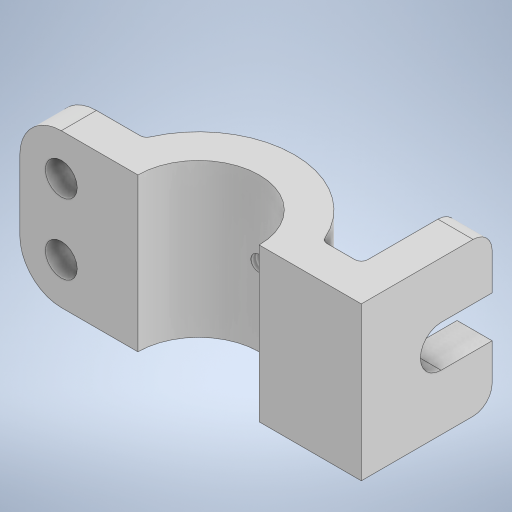
# Autodesk Inventor part: 3
Saved by Autodesk Inventor 2023 (Build 270158000, 158)
## iProperties
Created: 2023-10-10
Part Number: 3
Material: Všeobecné
Document SubType Name: Modeling
Designer: clu40164
Mass: 76.1606 g
Surface Area: 194.014 cm^2
Volume: 76.1606 cm^3
Density: 1 g/cm^3
Appearance: Výchozí
Author: clu40164
Autodesk Inventor part; units mm, degrees
ref_plane "YZ Plane" through (0, 0, 0) normal (1, 0, 0) x (0, 1, 0)
ref_plane "XZ Plane" through (0, 0, 0) normal (0, 1, 0) x (-1, 0, 0)
sketch "Náčrt1" plane through (0, 0, 0) normal (0, 1, 0) x (-1, 0, 0)
  arc A0 (-19, 0) -> (19, 0) centre (0, 0) ccw
  arc A1 (-27.4129, -12.1875) -> (27.4129, -12.1875) centre (0, 0) ccw
  line L0 (56, 0) -> (56, -11)
  line L1 (56, -11) -> (29.2404, -11)
  line L2 (-51, 0) -> (-51, -41)
  line L3 (-51, -41) -> (-40, -41)
  line L4 (-40, -41) -> (-40, -13)
  line L5 (-38, -11) -> (-29.2404, -11)
  arc A2 (29.2404, -11) -> (27.4129, -12.1875) centre (29.2404, -13) ccw
  arc A3 (-27.4129, -12.1875) -> (-29.2404, -11) centre (-29.2404, -13) ccw
  arc A4 (-38, -11) -> (-40, -13) centre (-38, -13) ccw
  line L6 (56, 0) -> (19, 0)
  line L7 (-19, 0) -> (-51, 0)
  point P0 (27.9106, -11)
  point P1 (-27.9106, -11)
  dimension "d0" = 19
  dimension "d1" = 30
  dimension "d3" = 107
  dimension "d4" = 51
  dimension "d5" = 11
  dimension "d6" = 41
  dimension "d7" = 11
  dimension "d8" = 2
  dimension "d9" = 2
  dimension "d10" = 2
  dimension "d16" = 96
  dimension "d17" = 56
  constraints: 16 end point, 12 point on circle, 8 tangent, 5 centre point, 3 perpendicular, 2 coincident, 2 point on line, 2 vertical, 1 collinear, 1 horizontal
  measures "d0" radius of A0
  measures "d1" radius of A1
  measures "d3" distance of L2.start L0.start
  measures "d4" distance of L2.start point (0, 0)
  measures "d5" distance of L0.start L0.end
  measures "d6" distance of L2.start L2.end
  measures "d7" distance of L2.end L3.end
  measures "d8" radius of A2
  measures "d9" radius of A3
  measures "d10" radius of A4
  measures "d16" distance between parallel lines of L4 L0
  measures "d17" distance from line of point (0, 0) L0
extrude "Vysunutí1" add sketch "Náčrt1" against normal blind 48
fillet "Zaoblení1" radius 13 1 edges at (-56, 0, -5.5)
fillet "Zaoblení2" radius 13 1 edges at (-56, -48, -5.5)
fillet "Zaoblení3" radius 6 2 edges at (45.5, -48, -41) (45.5, 0, -41)
sketch "Náčrt2" plane through (-29.2404, -48, -11) normal (0, 0, -1) x (-1, 0, 0)
  line L0 (-56.6532, 0) -> (-1.8275, 0) projected
  circle A0 centre (13.7596, 13) radius 5
  circle A1 centre (13.7596, 35) radius 5
  point P0 (-29.2404, 48)
  dimension "d26" = 10
  dimension "d27" = 10
  dimension "d28" = 35
  dimension "d29" = 13
  dimension "d30" = 38.3139
  dimension "d31" = 20.2968
  constraints: 2 centre point
  measures "d26" diameter of A0
  measures "d27" diameter of A1
  measures "d28" distance from line of A1.centre L0
  measures "d29" distance from line of A0.centre L0
  measures "d30" distance of L0.end A1.centre
  measures "d31" distance of L0.end A0.centre
extrude "Vysunutí2" cut sketch "Náčrt2" against normal blind 11
ref_plane "Pracovní rovina1" through (0, 0, -30) normal (0, 0, -1) x (-1, 0, 0)
sketch "Náčrt3" plane through (0, 0, -30) normal (0, 0, -1) x (-1, 0, 0)
  circle A0 centre (0, -24) radius 2.5
  point P0 (0, 0)
  dimension "d34" = 5
  constraints: 1 centre point
  measures "d34" diameter of A0
hole "Díra1" at (0, -24, -30) direction (0, 0, 1) diameter 4.9784 end through all thread size "1/4-20 UNC" class "2B" standard "ANSI Unified Screw Threads"
sketch "Náčrt4" plane through (51, -48, 0) normal (1, 0, 0) x (0, 0, -1)
  line L0 (0, 48) -> (0, 0) projected
  line L1 (0, 48) -> (35, 48) projected
  arc A0 (25, 30.5) -> (25, 17.5) centre (25, 24) ccw
  line L2 (25, 30.5) -> (41, 30.5)
  line L3 (25, 17.5) -> (41, 17.5)
  line L4 (41, 17.5) -> (41, 30.5)
  dimension "d45" = 13
  dimension "d46" = 24
  dimension "d47" = 25
  dimension "d48" = 41
  constraints: 6 end point, 2 horizontal, 2 point on circle, 2 tangent, 1 centre point, 1 perpendicular
  measures "d45" diameter of A0
  measures "d46" distance from line of A0.centre L1
  measures "d47" distance from line of A0.centre L0
  measures "d48" distance between parallel lines of L4 L0
extrude "Vysunutí3" cut sketch "Náčrt4" against normal blind 11
